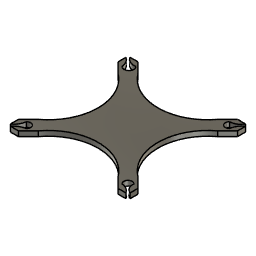
Drone_PCB (Autodesk Fusion 360 design; units mm, degrees)
Autodesk Fusion 360 part; units mm, degrees
sketch "Sketch1" plane through (0, 0, 0) normal (0, 0, 1) x (1, 0, 0)
  line L0 (50, -50) -> (-50, 50) construction
  line L1 (-50, -50) -> (50, 50) construction
  arc A0 (-50, -40) -> (-50, 40) centre (-80, 0) ccw
  arc A1 (40, -50) -> (-40, -50) centre (0, -80) ccw
  arc A2 (50, 40) -> (50, -40) centre (80, 0) ccw
  arc A3 (-40, 50) -> (40, 50) centre (0, 80) ccw
  line L2 (-50, 40) -> (-60, 50)
  line L3 (-50, 60) -> (-40, 50)
  line L4 (-50, -40) -> (-60, -50)
  line L5 (-50, -60) -> (-40, -50)
  line L6 (40, -50) -> (50, -60)
  line L7 (60, -50) -> (50, -40)
  line L8 (50, 40) -> (60, 50)
  line L9 (50, 60) -> (40, 50)
  arc A4 (48, 54) -> (58, 60) centre (48.1802, 65.033) ccw
  line L10 (46, 56) -> (56, 46) construction
  line L11 (-46, 56) -> (-57, 47) construction
  line L12 (-56, -46) -> (-46, -56) construction
  line L13 (56, -46) -> (46, -56) construction
  arc A5 (60, 58) -> (54, 48) centre (67.3571, 46.7857) ccw
  arc A6 (48, 54) -> (54, 48) centre (51, 51) ccw
  line L14 (60, 50) -> (60, 58)
  line L15 (58, 60) -> (50, 60)
  arc A7 (54, -48) -> (60, -58) centre (63.5909, -49.0455) ccw
  arc A8 (58, -60) -> (47.9908, -54.0092) centre (46.833, -67.3003) ccw
  arc A9 (54, -48) -> (47.9908, -54.0092) centre (50.9908, -51) ccw
  arc A10 (-48, -54) -> (-58, -60) centre (-45.5, -69.5) ccw
  arc A11 (-60, -58) -> (-54, -48) centre (-67.3571, -46.7857) ccw
  arc A12 (-48, -54) -> (-54, -48) centre (-51, -51) ccw
  arc A13 (-58, 60) -> (-47, 55) centre (-49, 65.2) ccw
  arc A14 (-54, 48) -> (-60, 58) centre (-67.3572, 46.7857) ccw
  arc A15 (-54, 48) -> (-47, 55) centre (-50.4048, 51.4048) ccw
  line L16 (-50, -60) -> (-58, -60)
  line L17 (-60, -58) -> (-60, -50)
  line L18 (58, -60) -> (50, -60)
  line L19 (60, -58) -> (60, -50)
  line L20 (-60, 50) -> (-60, 58)
  line L21 (-58, 60) -> (-50, 60)
  constraint coincident L0 origin
  constraint coincident L1 origin
  constraint parallel L2 L3
  constraint perpendicular L3 L4
  constraint parallel L4 L5
  constraint perpendicular L5 L6
  constraint parallel L6 L7
  constraint perpendicular L7 L8
  constraint parallel L8 L9
  constraint coincident L9 L10.start
  constraint coincident L8 L10.end
  constraint perpendicular L8 L10
  constraint coincident L3 L11.start
  constraint coincident L2 L11.end
  constraint coincident L4 L12.start
  constraint coincident L5 L12.end
  constraint perpendicular L5 L12
  constraint coincident L7 L13.start
  constraint coincident L6 L13.end
  constraint perpendicular L6 L13
  constraint coincident L10 A5.end
  constraint coincident L13 A7.start
  constraint coincident L13 A8.end
  constraint coincident L12 A10.start
  constraint coincident L12 A11.end
  constraint perpendicular L17 L18
extrude "Extrude1" add sketch "Sketch1" against normal blind 5
